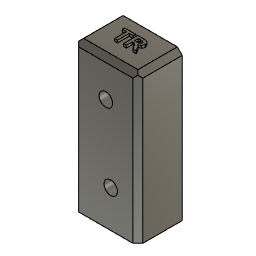
X#T8-Z_block_connector (Autodesk Fusion 360 design; units mm, degrees)
Autodesk Fusion 360 part; units mm, degrees
note: some values were not read from the file. Set by a fixed rule: which sketch regions a step uses.
sketch "Sketch1" plane through (0, 0, 0) normal (0, 0, 1) x (1, 0, 0)
  line L0 (0, 0) -> (30, 0)
  line L1 (30, 0) -> (30, 18)
  line L2 (30, 18) -> (0, 18)
  line L3 (0, 18) -> (0, 0)
  dimension "d1" = 30
  dimension "d2" = 18
  constraint horizontal L0
  constraint vertical L1
  constraint horizontal L2
  constraint vertical L3
  constraint coincident L0.start L3.end
  measures "d1" distance of L0.start L0.end
  measures "d2" distance of L0.start L2.end
extrude "Extrude1" add sketch "Sketch1" along normal blind 30
sketch "Sketch2" plane through (0, 18, 0) normal (0, 1, 0) x (-1, 0, 0)
  line L0 (-30, 0) -> (0, 0)
  line L1 (0, 0) -> (0, 30)
  line L2 (0, 30) -> (-30, 30)
  line L3 (-30, 30) -> (-30, 0)
  circle A0 centre (-15, 15) radius 2.75
  dimension "d5" = 5.5
  measures "d5" diameter of A0
extrude "Extrude2" cut sketch "Sketch2" against normal blind 46 contours A0
chamfer "Chamfer1" distance 3 angle 45 1 edges at (15, 0, 0)
extrude "Extrude3" add 1 faces at (10, 12, 30) along direction (0, 0, 1) blind 30
sketch "Sketch3" plane through (0, 0, 0) normal (0, -1, 0) x (1, 0, 0)
  line L0 (0, 3) -> (30, 3)
  line L1 (30, 3) -> (30, 60)
  line L2 (30, 60) -> (0, 60)
  line L3 (0, 60) -> (0, 3)
  circle A0 centre (15, 15) radius 2.75
  line L4 (15, 60) -> (15, 45)
  circle A1 centre (15, 45) radius 2.75
  dimension "d11" = 15
  dimension "d12" = 5.5
  constraint midpoint L2 L4.start
  constraint perpendicular L2 L4
  constraint coincident L4.end A1.centre
  measures "d11" distance of L4.start L4.end
  measures "d12" diameter of A1
extrude "Extrude4" cut sketch "Sketch3" against normal blind 50 contours A1
chamfer "Chamfer2" distance 3 angle 45 1 edges at (15, 0, 60)
chamfer "Chamfer3" distance 3 angle 45 2 edges at (0, 10.5, 60) (0, 0, 30)
chamfer "Chamfer4" distance 3 angle 45 2 edges at (30, 0, 30) (30, 10.5, 60)
sketch "Sketch4" plane through (0, 0, 0) normal (0, -1, 0) x (1, 0, 0)
  circle A0 centre (15, 45) radius 2.75
  circle A1 centre (15, 15) radius 2.75
  line L0 (27, 3) -> (27, 57)
  line L1 (27, 57) -> (3, 57)
  line L2 (3, 57) -> (3, 3)
  line L3 (3, 3) -> (27, 3)
  line L4 (10.8, 12.5751) -> (15, 10.1503)
  line L5 (15, 10.1503) -> (19.2, 12.5751)
  line L6 (19.2, 12.5751) -> (19.2, 17.4249)
  line L7 (19.2, 17.4249) -> (15, 19.8497)
  line L8 (15, 19.8497) -> (10.8, 17.4249)
  line L9 (10.8, 17.4249) -> (10.8, 12.5751)
  point P0 (15, 15)
  dimension "d18" = 4.2
  constraint coincident P0 A1.centre
  measures "d18" distance of P0 L9
extrude "Extrude5" cut sketch "Sketch4" against normal blind 5 contours L4 L5 L6 L7 L8 L9
chamfer "Chamfer5" distance 3 angle 45 2 edges at (30, 10.5, 0) (0, 10.5, 0)
delete_face "DeleteFace1" 1 faces at (2, 13, 1)
delete_face "DeleteFace2" 1 faces at (29, 13, 2)
delete_face "DeleteFace3" 1 faces at (19, 2, 1)
sketch "Sketch5" plane through (0, 0, 60) normal (0, 0, 1) x (-1, 0, 0)
  line L0 (-27, -3) -> (-27, -18)
  line L1 (-27, -18) -> (-3, -18)
  line L2 (-3, -18) -> (-3, -3)
  line L3 (-3, -3) -> (-27, -3)
  line L4 (-9.6342, -7.2242) -> (-20.06, -7.2242) construction
  line L5 (-20.06, -7.2242) -> (-20.06, -15.2242) construction
  line L6 (-20.06, -15.2242) -> (-9.6342, -15.2242) construction
  line L7 (-9.6342, -15.2242) -> (-9.6342, -7.2242) construction
  text T0 "TR" font "Arial" height 8 bold align ink ink in box 0 x 0 at (-9.6442, -7.2442) x (-1, 0) y (0, -1) spacing 1 height is em
  constraint perpendicular L4 L5
  constraint parallel L4 L6
  constraint parallel L5 L7
extrude "Extrude6" add sketch "Sketch5" along normal blind 1 text T0
sketch "Sketch6" plane through (0, 18, 0) normal (0, 1, 0) x (-1, 0, 0)
  line L0 (-30, 0) -> (0, 0)
  line L1 (0, 0) -> (0, 57)
  line L2 (0, 57) -> (-3, 60)
  line L3 (-3, 60) -> (-27, 60)
  line L4 (-27, 60) -> (-30, 57)
  line L5 (-30, 57) -> (-30, 0)
  circle A0 centre (-15, 15) radius 2.75
  circle A1 centre (-15, 45) radius 2.75
  line L6 (-19, 42.6906) -> (-15, 40.3812)
  line L7 (-15, 40.3812) -> (-11, 42.6906)
  line L8 (-11, 42.6906) -> (-11, 47.3094)
  line L9 (-11, 47.3094) -> (-15, 49.6188)
  line L10 (-15, 49.6188) -> (-19, 47.3094)
  line L11 (-19, 47.3094) -> (-19, 42.6906)
  point P0 (-15, 45)
  dimension "d24" = 4
  constraint coincident P0 A1.centre
  measures "d24" distance of P0 L11
extrude "Extrude7" cut sketch "Sketch6" against normal blind 4 contours L6 L7 L8 L9 L10 L11
sketch "Sketch7" plane through (0, 18, 0) normal (0, 1, 0) x (-1, 0, 0)
  line L0 (-15, 40.3812) -> (-19, 42.6906)
  line L1 (-19, 42.6906) -> (-19, 47.3094)
  line L2 (-19, 47.3094) -> (-15, 49.6188)
  line L3 (-15, 49.6188) -> (-11, 47.3094)
  line L4 (-11, 47.3094) -> (-11, 42.6906)
  line L5 (-11, 42.6906) -> (-15, 40.3812)
  line L6 (-30, 0) -> (0, 0)
  line L7 (0, 0) -> (0, 57)
  line L8 (0, 57) -> (-3, 60)
  line L9 (-3, 60) -> (-27, 60)
  line L10 (-27, 60) -> (-30, 57)
  line L11 (-30, 57) -> (-30, 0)
  circle A0 centre (-15, 15) radius 2.75
  line L12 (-20, 35) -> (-10, 35)
  line L13 (-10, 35) -> (-10, 23)
  line L14 (-10, 23) -> (-20, 23)
  line L15 (-20, 23) -> (-20, 35)
  line L16 (-10, 23) -> (-5, 23)
  line L17 (-5, 23) -> (-5, 35)
  line L18 (-5, 35) -> (-10, 35)
  line L19 (-10, 35) -> (-10, 23)
  line L20 (-20, 23) -> (-25, 23)
  line L21 (-25, 23) -> (-25, 35)
  line L22 (-25, 35) -> (-20, 35)
  line L23 (-20, 35) -> (-20, 23)
  constraint horizontal L12
  constraint vertical L13
  constraint horizontal L14
  constraint vertical L15
  constraint horizontal L16
  constraint vertical L17
  constraint horizontal L18
  constraint vertical L19
  constraint horizontal L20
  constraint vertical L21
  constraint horizontal L22
  constraint vertical L23
extrude "Extrude8" cut sketch "Sketch7" against normal blind 14 contours L12 L13 L14 L15 L19 L23 | L15 L20 L21 L22 L23 | L13 L16 L17 L18 L19
chamfer "Chamfer6" distance 1 angle 45 1 edges at (15, 4, 35)
extrude "Extrude9" add 1 faces at (13.1417, 5, 18.2187) along direction (0, -1, 0) blind 5
sketch "Sketch8" plane through (0, 0, 0) normal (0, -1, 0) x (1, 0, 0)
  circle A0 centre (15, 15) radius 2.75
  line L0 (3, 57) -> (3, 0)
  line L1 (3, 0) -> (27, 0)
  line L2 (27, 0) -> (27, 57)
  line L3 (27, 57) -> (3, 57)
  circle A1 centre (15, 45) radius 2.75
  circle A2 centre (15, 15) radius 2.75
  line L4 (0, 24) -> (96, 24)
  line L5 (48, 24) -> (17, 24)
  line L6 (17, 24) -> (17, 15)
  circle A3 centre (17, 15) radius 2.75
  dimension "d32" = 96
  dimension "d33" = 31
  dimension "d34" = 5.5
  constraint concentric A0 A2
  constraint perpendicular L2 L4
  constraint midpoint L4 L5.start
  constraint parallel L4 L5
  constraint perpendicular L5 L6
  constraint coincident L6.end A3.centre
  measures "d32" distance of L4.start L4.end
  measures "d33" distance of L5.start L5.end
  measures "d34" diameter of A3
extrude "Extrude10" add sketch "Sketch8" against normal blind 18 contours A0 A2 A3 picked at (13.6038, 14.7267)
extrude "Extrude11" cut sketch "Sketch8" against normal blind 18 contours A0 A2 L6 A3 | A0 A2 L6 A3
delete_face "DeleteFace4" 1 faces at (2, 1, 19)
delete_face "DeleteFace5" 1 faces at (1, 7, 58)
delete_face "DeleteFace6" 1 faces at (9, 1, 58)
delete_face "DeleteFace7" 1 faces at (28, 1, 39)
delete_face "DeleteFace8" 1 faces at (29, 6, 58)
extrude "Extrude12" cut 1 faces at (30, 6, 20) along direction (-1, 0, 0) blind 2
extrude "Extrude13" cut 1 faces at (0, 12, 20) along direction (1, 0, 0) blind 2
chamfer "Chamfer7" distance 2 angle 45 3 edges at (28, 9, 60) (15, 0, 60) (2, 9, 60)
chamfer "Chamfer8" distance 2 angle 45 2 edges at (28, 0, 29) (2, 0, 29)
sketch "Sketch9" plane through (0, 18, 0) normal (0, 1, 0) x (-1, 0, 0)
  line L0 (-2, 58) -> (-4, 60)
  line L1 (-4, 60) -> (-26, 60)
  line L2 (-26, 60) -> (-28, 58)
  line L3 (-28, 58) -> (-28, 0)
  line L4 (-28, 0) -> (-2, 0)
  line L5 (-2, 0) -> (-2, 58)
  line L6 (-5, 35) -> (-5, 23)
  line L7 (-5, 23) -> (-25, 23)
  line L8 (-25, 23) -> (-25, 35)
  line L9 (-25, 35) -> (-5, 35)
  line L10 (-15, 40.3812) -> (-19, 42.6906)
  line L11 (-19, 42.6906) -> (-19, 47.3094)
  line L12 (-19, 47.3094) -> (-15, 49.6188)
  line L13 (-15, 49.6188) -> (-11, 47.3094)
  line L14 (-11, 47.3094) -> (-11, 42.6906)
  line L15 (-11, 42.6906) -> (-15, 40.3812)
  circle A0 centre (-17, 15) radius 2.75
  line L16 (-21, 12.6906) -> (-17, 10.3812)
  line L17 (-17, 10.3812) -> (-13, 12.6906)
  line L18 (-13, 12.6906) -> (-13, 17.3094)
  line L19 (-13, 17.3094) -> (-17, 19.6188)
  line L20 (-17, 19.6188) -> (-21, 17.3094)
  line L21 (-21, 17.3094) -> (-21, 12.6906)
  point P0 (-17, 15)
  constraint coincident P0 A0.centre
extrude "Extrude14" cut sketch "Sketch9" against normal blind 4.5 contours L16 L17 L18 L19 L20 L21
sketch "Sketch10" plane through (0, 18, 0) normal (0, 1, 0) x (-1, 0, 0)
  line L0 (-17, 10.3812) -> (-21, 12.6906)
  line L1 (-21, 12.6906) -> (-21, 17.3094)
  line L2 (-21, 17.3094) -> (-17, 19.6188)
  line L3 (-17, 19.6188) -> (-13, 17.3094)
  line L4 (-13, 17.3094) -> (-13, 12.6906)
  line L5 (-13, 12.6906) -> (-17, 10.3812)
  line L6 (-2, 58) -> (-4, 60)
  line L7 (-4, 60) -> (-26, 60)
  line L8 (-26, 60) -> (-28, 58)
  line L9 (-28, 58) -> (-28, 0)
  line L10 (-28, 0) -> (-2, 0)
  line L11 (-2, 0) -> (-2, 58)
  line L12 (-5, 35) -> (-5, 23)
  line L13 (-5, 23) -> (-25, 23)
  line L14 (-25, 23) -> (-25, 35)
  line L15 (-25, 35) -> (-5, 35)
  line L16 (-15, 40.3812) -> (-19, 42.6906)
  line L17 (-19, 42.6906) -> (-19, 47.3094)
  line L18 (-19, 47.3094) -> (-15, 49.6188)
  line L19 (-15, 49.6188) -> (-11, 47.3094)
  line L20 (-11, 47.3094) -> (-11, 42.6906)
  line L21 (-11, 42.6906) -> (-15, 40.3812)
  line L22 (-21.15, 12.604) -> (-17, 10.208)
  line L23 (-17, 10.208) -> (-12.85, 12.604)
  line L24 (-12.85, 12.604) -> (-12.85, 17.396)
  line L25 (-12.85, 17.396) -> (-17, 19.792)
  line L26 (-17, 19.792) -> (-21.15, 17.396)
  line L27 (-21.15, 17.396) -> (-21.15, 12.604)
  point P0 (-17, 15)
  dimension "d47" = 4.15
  measures "d47" distance of P0 L27
extrude "Extrude15" cut sketch "Sketch10" against normal blind 4.5 contours L22 L23 L24 L25 L26 L27
